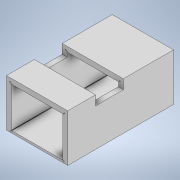
# Autodesk Inventor part: pyrodrone battery shield
Saved by Autodesk Inventor 2020 (Build 240168000, 168)
## iProperties
Created: 2021-05-15
Part Number: pyrodrone battery shield
Material: Generic
Document SubType Name: Modeling
Designer: Steven
Density: 1 g/cm^3
Appearance: Default
Author: Steven
Autodesk Inventor part; units mm, degrees
ref_plane "YZ Plane" through (0, 0, 0) normal (1, 0, 0) x (0, 1, 0)
ref_plane "XZ Plane" through (0, 0, 0) normal (0, 1, 0) x (-1, 0, 0)
ref_plane "XY Plane" through (0, 0, 0) normal (0, 0, 1) x (1, 0, 0)
sketch "Sketch1" plane through (0, 0, 0) normal (0, 1, 0) x (-1, 0, 0)
  line L0 (0, 0) -> (-50, 0)
  line L1 (-50, 0) -> (-50, -95)
  line L2 (-50, -95) -> (0, -95)
  line L3 (0, -95) -> (0, 0)
  dimension "d0" = 50
  dimension "d1" = 95
  constraints: 8 end point, 3 perpendicular, 1 horizontal
  measures "d0" distance of L0.start L0.end
  measures "d1" distance of L0.end L1.end
extrude "Extrusion1" add sketch "Sketch1" along normal blind 40
sketch "Sketch2" plane through (0, 0, 0) normal (0, 0, 1) x (1, 0, 0)
  line L0 (0, 0) -> (50, 0) construction
  line L1 (50, 0) -> (50, 40) construction
  line L2 (0, 40) -> (50, 40) construction
  line L3 (0, 0) -> (0, 40) construction
  line L4 (47.5, 37.5) -> (47.5, 2.5)
  line L5 (47.5, 2.5) -> (2.5, 2.5)
  line L6 (2.5, 2.5) -> (2.5, 37.5)
  line L7 (2.5, 37.5) -> (47.5, 37.5)
  dimension "d4" = 2.5
  dimension "d5" = 45
  dimension "d6" = 35
  constraints: 8 end point, 3 other
  measures "d4" distance between parallel lines of L2 L7
  measures "d5" distance of L6.end L4.start
  measures "d6" distance of L4.start L4.end
extrude "Extrusion2" cut sketch "Sketch2" against normal blind 90
sketch "Sketch3" plane through (0, 40, 0) normal (0, 1, 0) x (1, 0, 0)
  line L0 (50, 0) -> (50, 95) construction
  line L1 (50, 95) -> (0, 95) construction
  line L2 (0, 95) -> (0, 0) construction
  line L3 (0, 0) -> (50, 0) construction
  line L4 (50, 95) -> (0, 95) construction
  line L5 (25, 95) -> (25, 50) construction
  line L6 (25, 95) -> (25, 25) construction
  line L7 (25, 50) -> (50, 50)
  line L8 (50, 50) -> (50, 25)
  line L9 (50, 0) -> (50, 95) projected
  line L10 (50, 25) -> (0, 25)
  line L11 (0, 25) -> (0, 50)
  line L12 (0, 95) -> (0, 0) projected
  line L13 (0, 50) -> (25, 50)
  dimension "d9" = 45
  dimension "d10" = 70
  constraints: 14 end point, 5 point on line, 3 perpendicular, 2 vertical, 1 midpoint
  measures "d9" distance of L5.start L5.end
  measures "d10" distance of L5.start L6.end
extrude "Extrusion3" cut sketch "Sketch3" against normal blind 6
sketch "Sketch4" plane through (50, 0, -95) normal (0, 0, -1) x (-1, 0, 0)
  line L0 (0, 0) -> (50, 0) construction
  line L1 (50, 0) -> (50, 40) construction
  line L2 (0, 40) -> (50, 40) construction
  line L3 (0, 0) -> (0, 40) construction
  line L4 (0, 40) -> (50, 40) construction
  line L5 (25, 40) -> (25, 0) construction
  line L6 (50, 0) -> (0, 0) construction
  circle A0 centre (25, 20) radius 12.5
  dimension "d13" = 25
  constraints: 3 midpoint, 2 end point, 1 centre point
  measures "d13" diameter of A0
extrude "Extrusion4" cut sketch "Sketch4" against normal up to next
sketch "Sketch5" plane through (0, 0, -95) normal (-1, 0, 0) x (0, 0, 1)
  line L0 (45, 34) -> (45, 40) projected
  line L1 (0, 40) -> (45, 40) projected
  line L2 (0, 0) -> (0, 40) projected
  line L3 (0, 0) -> (95, 0) projected
  line L4 (95, 0) -> (95, 40) projected
  line L5 (70, 40) -> (95, 40) projected
  line L6 (70, 40) -> (70, 34) projected
  line L7 (70, 34) -> (45, 34) projected
extrude "Extrusion5" add sketch "Sketch5" along normal blind 2.5
sketch "Sketch6" plane through (50, 0, 0) normal (1, 0, 0) x (0, 0, -1)
  line L0 (50, 40) -> (50, 34) projected
  line L1 (50, 34) -> (25, 34) projected
  line L2 (25, 34) -> (25, 40) projected
  line L3 (0, 40) -> (25, 40) projected
  line L4 (0, 0) -> (0, 40) projected
  line L5 (0, 0) -> (95, 0) projected
  line L6 (95, 0) -> (95, 40) projected
  line L7 (50, 40) -> (95, 40) projected
extrude "Extrusion6" add sketch "Sketch6" along normal blind 2.5
sketch "Sketch7" plane through (0, 40, 0) normal (0, 1, 0) x (1, 0, 0)
  line L0 (-2.5, 25) -> (52.5, 25) projected
  line L1 (-2.5, 0) -> (-2.5, 25) projected
  line L2 (52.5, 0) -> (-2.5, 0) projected
  line L3 (52.5, 25) -> (52.5, 0) projected
  line L4 (-2.5, 50) -> (52.5, 50) projected
  line L5 (52.5, 95) -> (52.5, 50) projected
  line L6 (-2.5, 95) -> (52.5, 95) projected
  line L7 (-2.5, 50) -> (-2.5, 95) projected
  point P0 (0, 0)
extrude "Extrusion7" add sketch "Sketch7" along normal blind 2.5
sketch "Sketch10" plane through (-2.5, 0, 0) normal (0, 0, 1) x (1, 0, 0)
  line L0 (5, 2.5) -> (5, 37.5) projected
  line L1 (5, 37.5) -> (50, 37.5) projected
  line L2 (50, 37.5) -> (50, 2.5) projected
  line L3 (50, 2.5) -> (5, 2.5) projected
  line L4 (55, 0) -> (0, 0) projected
  line L5 (55, 0) -> (55, 42.5) projected
  line L6 (0, 42.5) -> (55, 42.5) projected
  line L7 (0, 0) -> (0, 42.5) projected
  line L8 (50.5, 38) -> (4.5, 38)
  line L9 (4.5, 38) -> (4.5, 2)
  line L10 (4.5, 2) -> (50.5, 2)
  line L11 (50.5, 2) -> (50.5, 38)
  point P0 (2.5, 0)
  dimension "d29" = 0.5
  constraints: 8 end point, 3 other
  measures "d29" distance between parallel lines of L1 L8
extrude "Extrusion9" cut sketch "Sketch10" against normal up to surface (90 mm away) contours L11 L10 L9 L8
sketch "Sketch11" plane through (-2.5, 0, 0) normal (0, 0, 1) x (1, 0, 0)
  line L0 (50.5, 38) -> (50.5, 2) projected
  line L1 (50.5, 2) -> (4.5, 2) projected
  line L2 (4.5, 2) -> (4.5, 38) projected
  line L3 (4.5, 38) -> (50.5, 38) projected
  line L4 (55, 0) -> (0, 0) projected
  line L5 (55, 0) -> (55, 42.5) projected
  line L6 (0, 42.5) -> (55, 42.5) projected
  line L7 (0, 0) -> (0, 42.5) projected
  line L8 (50.5, 38) -> (4.5, 38) projected
  arc A0 (4.3031, 38.1541) -> (4.3459, 37.8031) centre (4.5, 38) ccw construction
  line L9 (50.5, 2) -> (50.5, 38) projected
  arc A1 (4.3031, 1.8459) -> (4.6541, 1.8031) centre (4.5, 2) ccw construction
  line L10 (4.5, 38) -> (4.5, 2) construction
  line L11 (55, 41.5217) -> (4.5, 2) construction
  line L12 (0, 41.5217) -> (53.0556, 0) construction
  line L13 (4.5, 2) -> (1.9444, 0) construction
  line L14 (4.5, 38) -> (2.925, 39.2326) construction
  arc A2 (3.0791, 39.4295) -> (2.7709, 39.0357) centre (2.925, 39.2326) ccw
  line L15 (4.5, 2) -> (50.5, 2) construction
  line L16 (4.5, 2) -> (3.3187, 1.0755) construction
  arc A3 (3.5156, 1.2296) -> (3.1647, 1.2724) centre (3.3187, 1.0755) ccw construction
  line L17 (3.1647, 1.2724) -> (4.3459, 2.1969)
  line L18 (4.6541, 1.8031) -> (3.4728, 0.8787)
  arc A4 (4.3459, 2.1969) -> (4.3031, 1.8459) centre (4.5, 2) ccw construction
  arc A5 (4.6541, 1.8031) -> (4.3459, 2.1969) centre (4.5, 2) ccw construction
  arc A6 (3.4728, 0.8787) -> (3.5156, 1.2296) centre (3.3187, 1.0755) ccw construction
  arc A7 (3.1647, 1.2724) -> (3.4728, 0.8787) centre (3.3187, 1.0755) ccw
  line L19 (27.5, 38) -> (27.5, 2) construction
  line L20 (4.5, 2) -> (50.5, 2)
  line L21 (50.5, 2) -> (50.5, 38)
  line L22 (50.5, 38) -> (50.5, 2) construction
  line L23 (0, 41.5217) -> (50.5, 2) construction
  line L24 (50.5, 2) -> (53.0556, 0) construction
  line L25 (50.5, 2) -> (4.5, 2) construction
  line L26 (4.6541, 38.1969) -> (3.0791, 39.4295)
  line L27 (4.3459, 37.8031) -> (2.7709, 39.0357)
  arc A8 (3.1219, 39.0785) -> (3.0791, 39.4295) centre (2.925, 39.2326) ccw construction
  arc A9 (2.7709, 39.0357) -> (3.1219, 39.0785) centre (2.925, 39.2326) ccw construction
  arc A10 (4.6541, 38.1969) -> (4.3031, 38.1541) centre (4.5, 38) ccw construction
  arc A11 (4.3459, 37.8031) -> (4.6541, 38.1969) centre (4.5, 38) ccw construction
  circle A12 centre (5.1039, 37.5274) radius 0.25
  line L28 (4.6541, 38.1969) -> (5.258, 37.7243)
  line L29 (4.3459, 37.8031) -> (4.9498, 37.3305)
  circle A13 centre (5.1039, 2.4726) radius 0.25
  line L30 (4.3459, 2.1969) -> (4.9498, 2.6695)
  line L31 (4.6541, 1.8031) -> (5.258, 2.2757)
  arc A14 (50.6541, 37.8031) -> (50.6969, 38.1541) centre (50.5, 38) ccw construction
  arc A15 (50.3459, 1.8031) -> (50.6969, 1.8459) centre (50.5, 2) ccw construction
  line L32 (50.5, 38) -> (52.075, 39.2326) construction
  arc A16 (52.2291, 39.0357) -> (51.9209, 39.4295) centre (52.075, 39.2326) ccw
  line L33 (50.5, 2) -> (51.6813, 1.0755) construction
  arc A17 (51.8353, 1.2724) -> (51.4844, 1.2296) centre (51.6813, 1.0755) ccw construction
  line L34 (51.8353, 1.2724) -> (50.6541, 2.1969)
  line L35 (50.3459, 1.8031) -> (51.5272, 0.8787)
  arc A18 (50.6969, 1.8459) -> (50.6541, 2.1969) centre (50.5, 2) ccw construction
  arc A19 (50.6541, 2.1969) -> (50.3459, 1.8031) centre (50.5, 2) ccw construction
  arc A20 (51.4844, 1.2296) -> (51.5272, 0.8787) centre (51.6813, 1.0755) ccw construction
  arc A21 (51.5272, 0.8787) -> (51.8353, 1.2724) centre (51.6813, 1.0755) ccw
  line L36 (50.3459, 38.1969) -> (51.9209, 39.4295)
  line L37 (50.6541, 37.8031) -> (52.2291, 39.0357)
  arc A22 (51.9209, 39.4295) -> (51.8781, 39.0785) centre (52.075, 39.2326) ccw construction
  arc A23 (51.8781, 39.0785) -> (52.2291, 39.0357) centre (52.075, 39.2326) ccw construction
  arc A24 (50.6969, 38.1541) -> (50.3459, 38.1969) centre (50.5, 38) ccw construction
  arc A25 (50.3459, 38.1969) -> (50.6541, 37.8031) centre (50.5, 38) ccw construction
  circle A26 centre (49.8961, 37.5274) radius 0.25
  line L38 (50.3459, 38.1969) -> (49.742, 37.7243)
  line L39 (50.6541, 37.8031) -> (50.0502, 37.3305)
  circle A27 centre (49.8961, 2.4726) radius 0.25
  line L40 (50.6541, 2.1969) -> (50.0502, 2.6695)
  line L41 (50.3459, 1.8031) -> (49.742, 2.2757)
  point P0 (2.5, 0)
  point P1 (4.75, 2)
  point P2 (4.5, 2.25)
  point P3 (4.5, 37.75)
  point P4 (4.75, 38)
  point P5 (50.5, 2)
  dimension "d32" = 0.5
  dimension "d35" = 0.5
  dimension "d36" = 180
  dimension "d37" = 2
  dimension "d38" = 0.5
  dimension "d43" = 1.5
  dimension "d44" = 0.5
  dimension "d47" = 0.5
  dimension "d48" = 0.5
  constraints: 60 end point, 56 point on circle, 31 symmetric about line, 28 centre point, 19 point on line, 12 tangent, 9 coincident, 2 midpoint, 14 other
  measures "d32" diameter of A0
  measures "d35" diameter of A1
  measures "d36" angle of L11 L13
  measures "d37" distance of L14.start L14.end
  measures "d38" diameter of A2
  measures "d43" distance of L1.end L16.end
  measures "d44" diameter of A3
  measures "d47" diameter of A12
  measures "d48" diameter of A13
extrude "Extrusion10" cut sketch "Sketch11" against normal up to surface (90 mm away) contours L3 L38 L36 A16 L37 L39 L0 | L0 L39 A26 L38 L3 | L40 L34 A21 L35 L41 L1 L0 | L0 L1 L41 A27 L40 | L28 A12 L29 L2 L3 | L3 L2 L29 L27 A2 L26 L28 | L31 L18 A7 L17 L30 L2 L1 | L1 L2 L30 A13 L31
body "Solid1"
